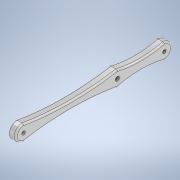
# Autodesk Inventor part: arm_34
Saved by Autodesk Inventor 2022 (Build 260153000, 153)
## iProperties
Created: 2024-10-19
Part Number: arm_34
Material: 一般
Document SubType Name: Modeling
Designer: acbaf
Density: 1 g/cm^3
Appearance: アルミニウム - ダーク
Author: acbaf
## iProperties of the stored document arm_54_3D プリント.ipt
Created: 2024-10-22
Part Number: arm_54_3D プリント
Material: 一般
Document SubType Name: Modeling
Designer: acbaf
Density: 1 g/cm^3
Appearance: 既定
Author: acbaf
Autodesk Inventor part; units mm, degrees
ref_plane "YZ Plane" through (0, 0, 0) normal (1, 0, 0) x (0, 1, 0)
ref_plane "XZ Plane" through (0, 0, 0) normal (0, 1, 0) x (-1, 0, 0)
ref_plane "XY Plane" through (0, 0, 0) normal (0, 0, 1) x (1, 0, 0)
sketch "スケッチ1" plane through (0, 0, 0) normal (1, 0, 0) x (0, 1, 0)
  circle A0 centre (3.839243, 0) radius 2.65
  circle A1 centre (3.839243, -60) radius 2.25
  circle A2 centre (3.839243, 120) radius 2.25
  circle A3 centre (3.839243, 120) radius 5
  circle A4 centre (3.839243, 0) radius 7.5
  circle A5 centre (3.839243, -60) radius 7.5
  line L0 (13.839243, -85.05003) -> (-6.160757, -85.05003)
  line L1 (-6.160757, -85.05003) -> (-6.160757, 157.537056)
  line L2 (-6.160757, 157.537056) -> (13.839243, 157.537056)
  line L3 (13.839243, 157.537056) -> (13.839243, -85.05003)
  arc A6 (13.839243, 140) -> (-6.160757, 140) centre (3.839243, 140) ccw
  arc A7 (-6.160757, -60) -> (13.839243, -60) centre (3.839243, -60) ccw
  arc A8 (-6.160757, -60) -> (-6.160757, 0) centre (-130.843864, -30) ccw
  line L4 (3.839243, 140) -> (3.839243, -60)
  arc A9 (13.839243, 0) -> (13.839243, -60) centre (138.52235, -30) ccw
  arc A10 (13.839243, 120) -> (-6.160757, 120) centre (3.839243, 120) ccw
  arc A11 (13.839243, 120) -> (13.839243, 0) centre (364.039727, 60) ccw
  arc A12 (-6.160757, 0) -> (-6.160757, 120) centre (-356.361242, 60) ccw
  point P0 (-6.160757, 0)
  dimension "d4" = 60
  dimension "d15" = 120
  dimension "d16" = 10
  dimension "d17" = 15
  dimension "d18" = 15
  dimension "d19" = 4.5
  dimension "d20" = 5.3
  dimension "d21" = 4.5
  dimension "d22" = 10
  dimension "d23" = 10
  constraints: 15 point on circle, 13 centre point, 10 end point, 8 point on line, 6 tangent, 4 symmetric about line, 3 coincident, 2 parallel, 1 horizontal, 1 perpendicular, 1 vertical, 2 other
  measures "d4" distance of A1.centre A0.centre
  measures "d15" distance of A2.centre A0.centre
  measures "d16" diameter of A3
  measures "d17" diameter of A4
  measures "d18" diameter of A5
  measures "d19" diameter of A2
  measures "d20" diameter of A0
  measures "d21" diameter of A1
  measures "d22" distance from line of L3 A0.centre
  measures "d23" distance from line of L1 A2.centre
extrude "押し出し2" add sketch "スケッチ1" along normal blind 10 contours A0 L4 A4 | A0 L4 A4 | A2 L4 A3 | A2 L4 A3 | A5 | A7 A8 A12 A10 A11 A9
fillet "フィレット3" radius 2 12 edges at (10, 8.7365, 60) (10, 3.8392, 130) (10, -1.058, 60) (10, -2.6024, -30) (10, 10.2809, -30) (10, 3.8392, -70) (0, 10.2809, -30) (0, 8.7365, 60) (0, 3.8392, 130) (0, 3.8392, -70) (0, -2.6024, -30) (0, -1.058, 60)
